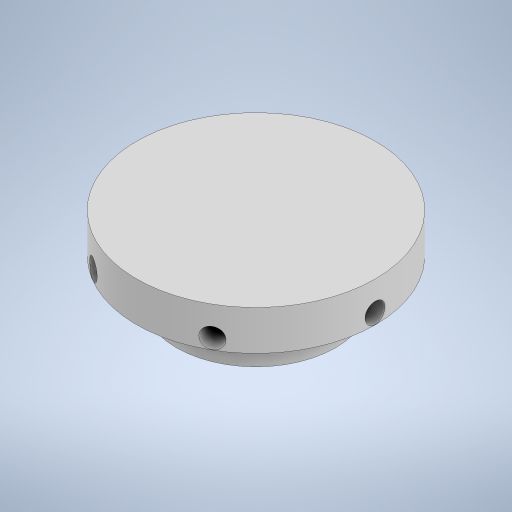
# Autodesk Inventor part: exp_tire_6rod_lower_rev0
Saved by Autodesk Inventor 2024 (Build 280153000, 153)
## iProperties
Created: 2024-04-09
Part Number: exp_tire_6rod_lower_rev0
Material: 一般
Document SubType Name: Modeling
Designer: Akio
Density: 1 g/cm^3
Appearance: 既定
Author: Akio
Autodesk Inventor part; units mm, degrees
ref_plane "YZ Plane" through (0, 0, 0) normal (1, 0, 0) x (0, 1, 0)
ref_plane "XZ Plane" through (0, 0, 0) normal (0, 1, 0) x (-1, 0, 0)
sketch "スケッチ1" plane through (0, 0, 0) normal (0, 1, 0) x (-1, 0, 0)
  circle A0 centre (0, 0) radius 10
  dimension "d0" = 20
  constraints: 1 centre point, 1 coincident
  measures "d0" diameter of A0
extrude "押し出し1" add sketch "スケッチ1" along normal blind 5
sketch "スケッチ2" plane through (0, 5, 0) normal (0, 1, 0) x (1, 0, 0)
  circle A0 centre (0, 0) radius 15
  dimension "dia_rod_base" = 30
  constraints: 1 centre point, 1 coincident
  measures "dia_rod_base" diameter of A0
extrude "押し出し2" add sketch "スケッチ2" along normal blind 5
sketch "スケッチ5" plane through (0, 0, 0) normal (0, -1, 0) x (1, 0, 0)
  line L0 (0, 1.5588) -> (1.35, 0.7794)
  line L1 (1.35, 0.7794) -> (1.35, -0.7794)
  line L2 (1.35, -0.7794) -> (0, -1.5588)
  line L3 (0, -1.5588) -> (-1.35, -0.7794)
  line L4 (-1.35, -0.7794) -> (-1.35, 0.7794)
  line L5 (-1.35, 0.7794) -> (0, 1.5588)
  point P0 (0, 0)
  point P1 (0, 0)
  dimension "d14" = 2.7
  constraints: 12 end point, 1 coincident, 13 other
  measures "d14" distance between parallel lines of L1 L4
extrude "押し出し3" cut sketch "スケッチ5" against normal blind 5
ref_plane "作業平面1" through (0, 0, 3) normal (0, 0, 1) x (1, 0, 0)
sketch "スケッチ10" plane through (0, 0, 3) normal (0, 0, 1) x (1, 0, 0)
  line L0 (15, 10) -> (-15, 10) projected
  line L1 (15, 10) -> (-15, 10) projected
  line L2 (15, 5) -> (-15.1085, 12.4268)
  line L3 (15, 5) -> (15, 10) projected
  line L4 (15, 5) -> (-15.1085, 12.4268)
  point P0 (0, 0)
  point P1 (0, 8.7)
  point P2 (0, 10)
  point P3 (-0.0543, 8.7134)
  dimension "d30" = 15
  dimension "d37" = 1.3
  constraints: 4 end point, 2 midpoint, 1 point on line
  measures "d30" distance from line of L3 point (0, 8.7)
  measures "d37" distance from line of L0 point (0, 8.7)
ref_plane "作業平面2" through (0, 8.7, 3) normal (-0.9877, -0.1564, 0) x (0, 0, 1)
sketch "スケッチ11" plane through (0, 8.7, 3) normal (-0.9877, -0.1564, 0) x (0, 0, 1)
  circle A0 centre (-3, 0) radius 1.25
  line L0 (-18, -3.6544) -> (-18, 1.284) projected
  line L1 (12, -3.6544) -> (12, 1.284) projected
  line L2 (-24, 0) -> (18, 0) projected
  point P0 (-3, -8.5929)
  dimension "d32" = 2.5
  dimension "d33" = 15
  constraints: 1 centre point, 1 midpoint
  measures "d32" diameter of A0
  measures "d33" distance from line of L0 A0.centre
extrude "押し出し6" cut sketch "スケッチ11" along normal through all
pattern_circular "円形状パターン2" count 6 over 360 about axis through (0, 5, 0) along (0, 1, 0) of "押し出し6"
equation "\"d30\" = 0.5 * dia_rod_base"
